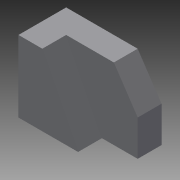
# Autodesk Inventor part: 7.1 Part 4
Saved by Autodesk Inventor 2015 (Build 190159000, 159)
## iProperties
Created: 2015-03-05
Part Number: 7.1 Part 4
Material: Generic
Document SubType Name: Modeling
Designer: PLTW-Stu-02
Density: 1 g/cm^3
Appearance: Default
Author: PLTW-Stu-02
Autodesk Inventor part; units mm, degrees
ref_plane "YZ Plane" through (0, 0, 0) normal (1, 0, 0) x (0, 1, 0)
ref_plane "XZ Plane" through (0, 0, 0) normal (0, 1, 0) x (-1, 0, 0)
ref_plane "XY Plane" through (0, 0, 0) normal (0, 0, 1) x (1, 0, 0)
sketch "Sketch1" plane through (0, 0, 0) normal (0, 0, 1) x (1, 0, 0)
  line L0 (11.6217, 9.037) -> (62.4217, 9.037)
  line L1 (62.4217, 9.037) -> (62.4217, 47.137)
  line L2 (62.4217, 47.137) -> (11.6217, 47.137)
  line L3 (11.6217, 47.137) -> (11.6217, 9.037)
  point P0 (0, 0)
  point P1 (24.3217, 47.137)
  dimension "d0" = 50.8
  dimension "d1" = 38.1
  dimension "d2" = 12.7
  constraints: 8 end point, 2 parallel, 1 horizontal, 1 perpendicular, 1 point on line
  measures "d0" distance of L2.end L1.end
  measures "d1" distance of L1.end L0.end
  measures "d2" distance from line of L3 point (24.322, 47.137)
extrude "Extrusion1" add sketch "Sketch1" along normal blind 25.4
sketch "Sketch2" plane through (0, 0, 25.4) normal (0, 0, 1) x (1, 0, 0)
  line L0 (24.3217, 47.137) -> (43.3717, 9.037)
  line L1 (24.3217, 47.137) -> (62.4217, 47.137)
  line L2 (62.4217, 47.137) -> (62.4217, 9.037)
  line L3 (62.4217, 9.037) -> (62.4217, 47.137) projected
  line L4 (62.4217, 9.037) -> (43.3717, 9.037)
  point P0 (0, 0)
  constraints: 8 end point, 1 collinear, 1 horizontal, 1 perpendicular
extrude "Extrusion2" cut sketch "Sketch2" against normal blind 12.7
sketch "Sketch3" plane through (0, 0, 12.7) normal (0, 0, 1) x (1, 0, 0)
  line L0 (49.7217, 47.137) -> (62.4217, 28.087)
  line L1 (49.7217, 47.137) -> (62.4217, 47.137)
  line L2 (62.4217, 47.137) -> (62.4217, 28.087)
  point P0 (0, 0)
  constraints: 6 end point, 1 horizontal, 1 perpendicular
extrude "Extrusion3" cut sketch "Sketch3" against normal blind 12.7
body "Solid1"
